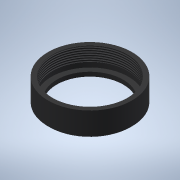
# Autodesk Inventor part: Überwurfmutter
Saved by Autodesk Inventor 2020.2 (Build 242310000, 310)
## iProperties
Part Number: Überwurfmutter
Document SubType Name: Modellieren
Density: 0.357273 g/cm^3
Material: PC/ABS-Kunststoff
Appearance: Dunkelgrau
Mass: 4.00806 g
Surface Area: 86.1837 cm^2
Volume: 11.2185 cm^3
Sheet Metal Rule: Standard
Created: 2020-10-30
Control State: 0
Master: False
Checked Out: False
Shininess: 64.0
Length Units: 11269
Angle Units: 11279
Time Units: 11290
Mass Units: 11283
Length Display Precision: 3
Angle Display Precision: 2
Compacted: True
Density: 0.0
Volumn: 0.0
Area: 0.0
PropertySet Name: Model Information
Autodesk Inventor part; units mm, degrees
ref_plane "YZ Plane" through (0, 0, 0) normal (1, 0, 0) x (0, 1, 0)
sketch "Skizze2" plane through (0, 0, 0) normal (0, 0, 1) x (1, 0, 0)
  circle A0 centre (0, 0) radius 30
  dimension "d0" = 60
  constraints: 1 centre point, 1 coincident
  measures "d0" diameter of A0
extrude "Extrusion1" add sketch "Skizze2" along normal blind 17
sketch "Skizze8" plane through (0, 0, 17) normal (0, 0, 1) x (1, 0, 0)
  circle A0 centre (0, 0) radius 30 projected
  constraints: 1 coincident
hole "Bohrung1" at (0, 0, 17) direction (0, 0, -1) diameter 47.5 end through all
ref_plane "Arbeitsebene1" through (0, 0, 3) normal (0, 0, -1) x (-1, 0, 0)
ref_plane "Arbeitsebene2" through (0, 0, 7) normal (0, 0, -1) x (-1, 0, 0)
sketch "Skizze6" plane through (0, 0, 17) normal (0, 0, 1) x (1, 0, 0)
  circle A0 centre (0, 0) radius 23.75 projected
  circle A1 centre (0, 0) radius 30 projected
  circle A2 centre (0, 0) radius 27.5
  dimension "d34" = 55
  constraints: 1 centre point, 1 coincident
  measures "d34" diameter of A2
extrude "Extrusion4" cut sketch "Skizze6" against normal up to surface (4 mm away) from surface at -10 contours A2
sketch "Skizze7" plane through (0, 0, 17) normal (0, 0, 1) x (1, 0, 0)
  circle A0 centre (0, 0) radius 30 projected
  constraints: 1 coincident
hole "Bohrung2" at (0, 0, 17) direction (0, 0, -1) diameter 53.5 depth 10 tip angle 118
thread "Gewinde3" size "M55x1.5" class "6H" standard "ANSI Metric M Profile" length 10
chamfer "Fase4" distance 1 angle 45 1 edges at (-30, 0, 0)
sketch "Skizze9" plane through (0, 0, 0) normal (0, 0, -1) x (-1, 0, 0)
  point P0 (0, 0)
  point P1 (23.75, 0)
  dimension "d51" = 23.75
  constraints: 1 horizontal alignment
  measures "d51" distance of point (0, 0) point (23.75, 0)
hole "Bohrung3" at (-23.75, 0, 0) direction (0, 0, 1) diameter 6 end through all
equation "\"Biegeradius\" = Stärke"
equation "\"BreiteBiegungsfreistellung\" = Stärke"
equation "\"TiefeBiegungsfreistellung\" = 0.5 * Stärke"
equation "\"GrößeEckenfreistellung\" = 4 * Stärke"
equation "\"MinimalRest\" = 2 * Stärke"
equation "\"Übergangsradius\" = Biegeradius"
equation "\"JacobiRadiusGröße\" = Stärke"
equation "\"Abstandsgröße\" = Stärke"
equation "\"Stärke\" = 0.5"
